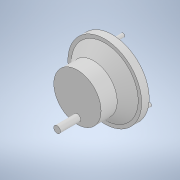
# Autodesk Inventor part: MPG
Saved by Autodesk Inventor 2022 (Build 260153000, 153)
## iProperties
Created: 2022-10-09
Part Number: MPG
Material: Generic
Document SubType Name: Modeling
Designer: Nick
Density: 1 g/cm^3
Appearance: Default
Author: Nick
Autodesk Inventor part; units mm, degrees
ref_plane "YZ Plane" through (0, 0, 0) normal (1, 0, 0) x (0, 1, 0)
ref_plane "XZ Plane" through (0, 0, 0) normal (0, 1, 0) x (-1, 0, 0)
ref_plane "XY Plane" through (0, 0, 0) normal (0, 0, 1) x (1, 0, 0)
sketch "Sketch1" plane through (0, 0, 0) normal (0, 0, 1) x (1, 0, 0)
  circle A0 centre (0, 0) radius 30.099
  dimension "d0" = 60.198
  constraints: 1 centre point, 1 coincident
  measures "d0" diameter of A0
extrude "Extrusion1" add sketch "Sketch1" along normal blind 6.1468
sketch "Sketch2" plane through (0, 0, 0) normal (0, 0, -1) x (-1, 0, 0)
  circle A0 centre (0, 0) radius 21.3106
  dimension "d3" = 42.6212
  constraints: 1 centre point, 1 coincident
  measures "d3" diameter of A0
extrude "Extrusion2" add sketch "Sketch2" along normal blind 5.08
sketch "Sketch3" plane through (0, 0, 0) normal (0, 0, -1) x (-1, 0, 0)
  circle A0 centre (0, 0) radius 21.3106 projected
  circle A1 centre (0, 0) radius 30.099 projected
  line L0 (0, 25.4139) -> (22.0091, -12.707) construction
  line L1 (22.0091, -12.707) -> (-22.0091, -12.707) construction
  line L2 (-22.0091, -12.707) -> (0, 25.4139) construction
  circle A2 centre (0, 25.4139) radius 1.4224
  circle A3 centre (22.0091, -12.707) radius 1.4224
  circle A4 centre (-22.0091, -12.707) radius 1.4224
  line L3 (-11.071, 20.6645) -> (5.4814, 30.221) construction
  line L4 (36.2551, -6.1245) -> (10.9127, -20.7559) construction
  dimension "d6" = 44.0182
  dimension "d7" = 2.8448
  dimension "d8" = 46.863
  constraints: 10 end point, 4 coincident, 3 centre point, 2 equal radius, 2 tangent, 1 horizontal, 1 parallel, 1 perpendicular, 7 other
  measures "d6" distance of L0.start L0.end
  measures "d7" diameter of A2
  measures "d8" distance between parallel lines of L4 L3
extrude "Extrusion3" add sketch "Sketch3" along normal blind 8.6868 contours A2 | A3 | A4
sketch "Sketch4" plane through (0, 0, 0) normal (1, 0, 0) x (0, 1, 0)
  line L0 (30.099, 6.1468) -> (-30.099, 6.1468) projected
  line L1 (27.2941, 6.1468) -> (19.2856, 15.3189)
  line L2 (19.2856, 15.3189) -> (19.2856, 28.4756)
  line L3 (19.2856, 28.4756) -> (0, 28.4756)
  line L4 (0, 28.4756) -> (0, 0)
  point P0 (0, 6.1468)
  constraints: 8 end point, 2 perpendicular, 1 point on line, 1 vertical
revolve "Revolution1" add sketch "Sketch4" angle 360 about axis through (0, 0, 28.4756) along (0, 0, -1)
sketch "Sketch5" plane through (0, 0, 28.4756) normal (0, 0, 1) x (1, 0, 0)
  circle A0 centre (0, -14.4677) radius 2.7154
  point P0 (0, 0)
  constraints: 1 centre point
extrude "Extrusion4" add sketch "Sketch5" along normal blind 16.6243
body "Solid1"
